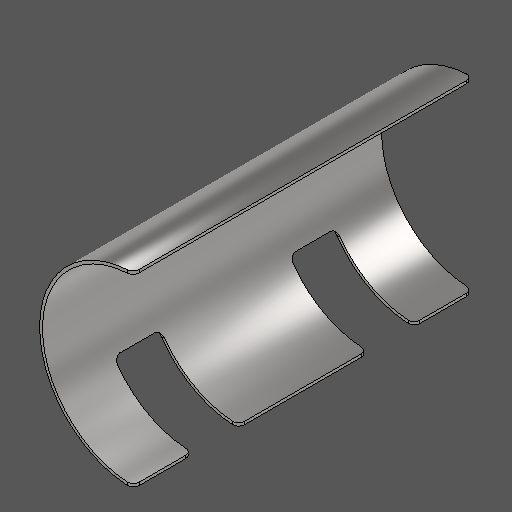
# Autodesk Inventor part: LP-screen-sheet-metal
Saved by Autodesk Inventor 2025 (Build 290162000, 162)
## iProperties
Created: 2024-06-05
Part Number: LP-screen-sheet-metal
Material: Stainless Steel
Document SubType Name: Sheet Metal
Designer: kuzmin
Density: 8 g/cm^3
Sheet Metal Rule: Default_mm
Appearance: Semi-Polished
Flat Pattern Width: 5.8 cm
Flat Pattern Length: 4.93858 cm
Flat Pattern Area: 28.6438 cm^2
Sheet Metal Width: 58,000 mm
Sheet Metal Length: 49,386 mm
Sheet Metal Area: 2864,379 mm^2
Author: kuzmin
Autodesk Inventor part; units mm, degrees
ref_plane "YZ Plane" through (0, 0, 0) normal (1, 0, 0) x (0, 1, 0)
ref_plane "XZ Plane" through (0, 0, 0) normal (0, 1, 0) x (-1, 0, 0)
ref_plane "XY Plane" through (0, 0, 0) normal (0, 0, 1) x (1, 0, 0)
sketch "Sketch1" plane through (0, 0, 0) normal (0, 0, 1) x (1, 0, 0)
  circle A0 centre (0, 0) radius 15.5
  circle A1 centre (0, 0) radius 16
  dimension "d0" = 32
  dimension "d1" = 0.5
  constraints: 2 centre point, 2 coincident
  measures "d0" diameter of A1
  measures "d1" radial gap between concentric circles of A1 A0
extrude "Extrusion1" add sketch "Sketch1" along normal mid plane 58
sketch "Sketch3" plane through (0, 0, 29) normal (0, 0, 1) x (1, 0, 0)
  circle A0 centre (0, 0) radius 15.5 construction
  circle A1 centre (0, 0) radius 16 construction
  line L0 (0, -20) -> (20, -20)
  line L1 (20, -20) -> (20, 20)
  line L2 (20, 20) -> (0, 20)
  line L3 (0, 20) -> (0, -20)
  dimension "d8" = 20
  dimension "d9" = 40
  constraints: 8 end point, 2 parallel, 1 coincident, 1 horizontal, 1 midpoint, 1 perpendicular
  measures "d8" distance of L1.end L2.end
  measures "d9" distance of L0.end L1.end
extrude "Extrusion3" cut sketch "Sketch3" against normal through all
sketch "Sketch4" plane through (0, 0, 0) normal (1, 0, 0) x (0, 1, 0)
  line L0 (-18, -19) -> (-8, -19)
  line L1 (-8, -19) -> (-8, -11)
  line L2 (-8, -11) -> (-18, -11)
  line L3 (-18, -11) -> (-18, -19)
  line L4 (-16, -29) -> (16, -29) projected
  line L5 (-16, -29) -> (-16, 29) projected
  point P0 (0, 0)
  dimension "d12" = 8
  dimension "d13" = 10
  dimension "d14" = 2
  dimension "d17" = 8
  constraints: 8 end point, 2 parallel, 1 horizontal, 1 perpendicular
  measures "d12" distance of L2.end L0.start
  measures "d13" distance between parallel lines of L4 L0
  measures "d14" distance between parallel lines of L5 L3
  measures "d17" distance between parallel lines of L1 L5
extrude "Extrusion4" cut sketch "Sketch4" against normal through all
mirror "Mirror1" about plane through (0, 0, 0) normal (0, 0, 1) of "Extrusion4"
fillet "Fillet1" radius 1 12 edges at (0, -15.75, 19) (0, -15.75, 11) (0, -15.75, 29) (0, 15.75, 29) (-13.5662, -8, 19) (-13.5662, -8, 11) (-13.5662, -8, -11) (0, -15.75, -11) (-13.5662, -8, -19) (0, -15.75, -19) (0, -15.75, -29) (0, 15.75, -29)
body "Solid1"
